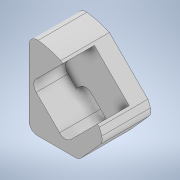
# Autodesk Inventor part: BatterySwitchHolder
Saved by Autodesk Inventor 2020 (Build 240168000, 168)
## iProperties
Created: 2020-09-16
Part Number: BatterySwitchHolder
Material: Generic
Document SubType Name: Modeling
Designer: kstrm-adm
Density: 1 g/cm^3
Appearance: Default
Author: kstrm-adm
Autodesk Inventor part; units mm, degrees
ref_plane "YZ Plane" through (0, 0, 0) normal (1, 0, 0) x (0, 1, 0)
ref_plane "XZ Plane" through (0, 0, 0) normal (0, 1, 0) x (-1, 0, 0)
ref_plane "XY Plane" through (0, 0, 0) normal (0, 0, 1) x (1, 0, 0)
sketch "Sketch1" plane through (0, 0, 0) normal (0, 0, 1) x (1, 0, 0)
  line L0 (0, -52.8422) -> (0, 52.8422) projected
  line L1 (-52.8422, 0) -> (52.8422, 0) projected
  circle A0 centre (0, 0) radius 37.7444
  line L2 (0, 37.7444) -> (0, 0)
  line L3 (0, 0) -> (37.7444, 0)
  circle A1 centre (0, 0) radius 30.1244
  line L4 (0, 0) -> (29.0087, 8.1224)
  line L5 (12.3571, 27.4733) -> (27.455, 12.3976)
  line L6 (29.0087, 8.1224) -> (21.7807, 0)
  point P0 (0, 30.1244)
  dimension "d0" = 75.4888
  dimension "d1" = 7.62
  dimension "d2" = 21.336
  dimension "d3" = 12.3571
  constraints: 10 end point, 5 point on circle, 3 point on line, 2 centre point, 1 coincident, 1 collinear
  measures "d0" diameter of A0
  measures "d1" radial gap between concentric circles of A0 A1
  measures "d2" distance of L5.start L5.end
  measures "d3" distance from line of L5.start L2
extrude "Extrusion1" add sketch "Sketch1" along normal blind 19.05 contours L4 L6 L1 | L0 A1 L5 L4
sketch "Sketch2" plane through (12.3571, 27.4733, 19.05) normal (0.7065855, 0.7076277, 0) x (0.7076277, -0.7065855, 0)
  line L0 (21.336, 0) -> (0, 0) projected
  line L1 (1.016, 0) -> (20.32, 0)
  line L2 (20.32, 0) -> (20.32, 12.446)
  line L3 (20.32, 12.446) -> (1.016, 12.446)
  line L4 (1.016, 12.446) -> (1.016, 0)
  line L5 (0, 19.05) -> (0, 0) projected
  point P0 (10.668, 19.05)
  dimension "d6" = 19.304
  dimension "d7" = 12.446
  dimension "d8" = 1.016
  constraints: 8 end point, 2 parallel, 1 horizontal, 1 perpendicular, 1 point on line
  measures "d6" distance of L3.end L2.end
  measures "d7" distance of L3.end L1.start
  measures "d8" distance between parallel lines of L5 L4
extrude "Extrusion2" cut sketch "Sketch2" against normal blind 17.78
move faces "Move1" translate (0, -2.54, 0) faces at (7.2602, 0, 6.35)
sketch "Sketch3" plane through (13.076, 26.7554, 6.604) normal (0, 0, 1) x (0.7076277, -0.7065855, 0)
  line L0 (19.304, -17.78) -> (0, -17.78) projected
  line L1 (19.304, -17.78) -> (7.874, -17.78)
  line L2 (7.874, -17.78) -> (7.874, -12.7)
  line L3 (7.874, -12.7) -> (19.304, -12.7)
  line L4 (19.304, -12.7) -> (19.304, -17.78)
  point P0 (9.652, -28.1722)
  point P1 (7.874, -17.78)
  dimension "d14" = 11.43
  dimension "d15" = 5.08
  constraints: 8 end point, 2 parallel, 1 horizontal, 1 perpendicular
  measures "d14" distance of L2.end L3.end
  measures "d15" distance of L1.end L2.end
extrude "Extrusion3" cut sketch "Sketch3" against normal blind 19.05
fillet "Fillet1" radius 3.175 9 edges at (0.5115, 14.1724, 12.827) (14.1716, 0.5324, 12.827) (14.1723, 0.5331, 6.604) (14.173, 0.5339, 3.302) (0, -2.54, 9.525) (0, 30.1244, 9.525) (19.5204, -2.54, 9.525) (29.0087, 8.1224, 9.525) (9.6743, 12.2049, 3.302)
body "Solid1"
